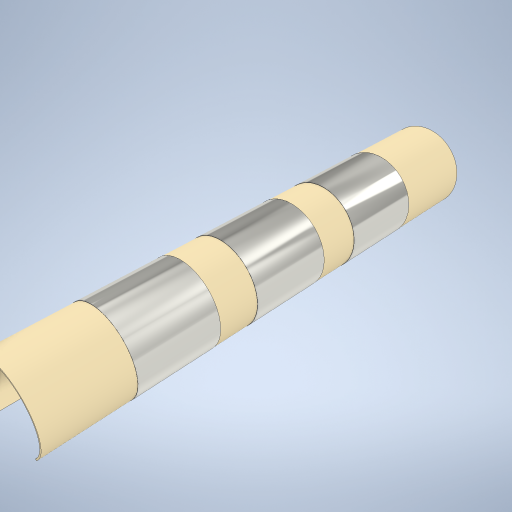
# Autodesk Inventor part: Cano
Saved by Autodesk Inventor 2024.4 (Build 284460000, 460)
## iProperties
Created: 2026-08-16
Part Number: Cano
Material: Generic
Document SubType Name: Modeling
Designer: MaryPinkAssus
Density: 1 g/cm^3
Appearance: Default
Author: MaryPinkAssus
Autodesk Inventor part; units mm, degrees
ref_plane "YZ Plane" through (0, 0, 0) normal (1, 0, 0) x (0, 1, 0)
ref_plane "XZ Plane" through (0, 0, 0) normal (0, 1, 0) x (-1, 0, 0)
ref_plane "XY Plane" through (0, 0, 0) normal (0, 0, 1) x (1, 0, 0)
sketch "Base" plane through (0, 0, 0) normal (0, 0, 1) x (1, 0, 0)
  circle A0 centre (0, 0) radius 25
  circle A1 centre (0, 0) radius 26
  line L0 (0, 0) -> (-18.3848, -18.3848)
  line L1 (0, -36.4) -> (0, 36.4) construction
  line L2 (0, 0) -> (18.3848, -18.3848)
  point P0 (17.6777, -17.6777)
  point P1 (18.3848, -18.3848)
  point P2 (-17.6777, -17.6777)
  dimension "d1" = 52
  dimension "d0" = 50
  dimension "d4" = 45
  constraints: 4 end point, 2 coincident, 1 centre point, 1 symmetric about line, 3 other
  measures "d0" diameter of A0
  measures "d4" angle of L1 L0
extrude "Corpo" add sketch "Base" along normal blind 300 contours A0 L0 A1 L2 picked at (-19.4545, -16.4764)
sketch "FolhaAluminio" plane through (-17.6777, -17.6777, 300) normal (0.7071068, -0.7071068, 0) x (-0.7071068, -0.7071068, 0)
  line L0 (-51, 300) -> (1, 300) projected
  line L1 (1, 300) -> (1, 250) construction
  line L2 (1, 300) -> (1, 0) projected
  line L3 (1, 250) -> (1.2, 250)
  line L4 (1.2, 250) -> (1.2, 200)
  line L5 (1.2, 200) -> (1, 200)
  line L6 (1, 200) -> (1, 250)
  line L7 (1, 200) -> (1, 175) construction
  line L8 (1, 175) -> (1.2, 175)
  line L9 (1.2, 175) -> (1.2, 125)
  line L10 (1.2, 125) -> (1, 125)
  line L11 (1, 125) -> (1, 175)
  line L12 (1, 125) -> (1, 100) construction
  line L13 (1, 100) -> (1.2, 100)
  line L14 (1.2, 100) -> (1.2, 50)
  line L15 (1.2, 50) -> (1, 50)
  line L16 (1, 50) -> (1, 100)
  line L17 (-25, 360) -> (-25, -60) projected
  point P0 (-25, 300)
  point P1 (1, 200)
  point P2 (1, 125)
  point P3 (1, 50)
  dimension "d5" = 50
  dimension "d6" = 0.2
  dimension "d7" = 50
  dimension "d8" = 25
  dimension "d9" = 0.2
  dimension "d10" = 50
  dimension "d11" = 25
  dimension "d12" = 0.2
  dimension "d13" = 50
  constraints: 30 end point, 6 parallel, 3 horizontal, 3 perpendicular, 3 point on line
  measures "d5" distance of L0.end L1.end
  measures "d6" distance of L4.end L5.end
  measures "d7" distance of L3.end L4.end
  measures "d8" distance of L5.end L7.end
  measures "d9" distance of L9.end L10.end
  measures "d10" distance of L8.end L9.end
  measures "d11" distance of L10.end L12.end
  measures "d12" distance of L14.end L15.end
  measures "d13" distance of L13.end L14.end
revolve "Folhas" add sketch "FolhaAluminio" angle 270 about axis through (0, 0, -10) along (0, 0, -1) separate body
body "Solid1"
body "Solid2"
